Autodesk Fusion 360 part; units mm, degrees
(part 11 of 14)
  spline S137 degree 5 poles (-10.4982, 16.1129) (-10.4995, 16.1142) (-10.5054, 16.12) (-10.516, 16.1305) (-10.5314, 16.1454) (-10.5515, 16.1648) (-10.5752, 16.1872) (-10.5991, 16.2096) (-10.6232, 16.2317) (-10.6474, 16.2537) (-10.6718, 16.2756) (-10.6964, 16.2974) (-10.7212, 16.319) (-10.7461, 16.3405) (-10.7712, 16.3619) (-10.7965, 16.3832) (-10.8219, 16.4043) (-10.8474, 16.4253) (-10.8731, 16.4462) (-10.899, 16.4669) (-10.925, 16.4876) (-10.9511, 16.5081) (-10.9774, 16.5286) (-11.0038, 16.5489) (-11.0303, 16.5691) (-11.057, 16.5891) (-11.0838, 16.6091) (-11.1108, 16.629) (-11.1378, 16.6487) (-11.165, 16.6684) (-11.1924, 16.6879) (-11.2198, 16.7073) (-11.2474, 16.7267) (-11.2751, 16.7459) (-11.3029, 16.765) (-11.3308, 16.784) (-11.3589, 16.8029) (-11.387, 16.8217) (-11.4153, 16.8404) (-11.4437, 16.859) (-11.4722, 16.8775) (-11.5008, 16.8959) (-11.5295, 16.9142) (-11.5584, 16.9324) (-11.5873, 16.9505) (-11.6163, 16.9685) (-11.6455, 16.9864) (-11.6748, 17.0042) (-11.7041, 17.0219) (-11.7336, 17.0395) (-11.7632, 17.057) (-11.7928, 17.0744) (-11.8226, 17.0917) (-11.8525, 17.1089) (-11.8824, 17.126) (-11.9125, 17.143) (-11.9427, 17.1599) (-11.9729, 17.1768) (-11.9972, 17.1902) (-12.0155, 17.2001) (-12.0277, 17.2068) (-12.0338, 17.2101) knots 0.195913 0.195913 0.195913 0.195913 0.195913 0.195913 0.2 0.214286 0.228571 0.242857 0.257143 0.271429 0.285714 0.3 0.314286 0.328571 0.342857 0.357143 0.371429 0.385714 0.4 0.414286 0.428571 0.442857 0.457143 0.471429 0.485714 0.5 0.514286 0.528571 0.542857 0.557143 0.571429 0.585714 0.6 0.614286 0.628571 0.642857 0.657143 0.671429 0.685714 0.7 0.714286 0.728571 0.742857 0.757143 0.771429 0.785714 0.8 0.814286 0.828571 0.842857 0.857143 0.871429 0.885714 0.9 0.914286 0.928571 0.942857 0.957143 0.971429 0.985714 1 1 1 1 1 1
  arc A69 (-12.0338, 17.2101) -> (-12.6491, 16.763) centre (0, 0) ccw
  spline S138 degree 5 poles (-12.6491, 16.763) (-12.6479, 16.7562) (-12.6453, 16.7426) (-12.6415, 16.7221) (-12.6362, 16.6949) (-12.6296, 16.6609) (-12.6228, 16.627) (-12.6159, 16.5931) (-12.6089, 16.5593) (-12.6018, 16.5256) (-12.5945, 16.4919) (-12.5871, 16.4583) (-12.5796, 16.4248) (-12.572, 16.3913) (-12.5642, 16.3579) (-12.5563, 16.3246) (-12.5483, 16.2913) (-12.5402, 16.2582) (-12.5319, 16.225) (-12.5235, 16.192) (-12.515, 16.159) (-12.5064, 16.1261) (-12.4976, 16.0933) (-12.4887, 16.0606) (-12.4796, 16.0279) (-12.4704, 15.9953) (-12.4611, 15.9628) (-12.4517, 15.9303) (-12.4421, 15.898) (-12.4324, 15.8657) (-12.4225, 15.8335) (-12.4125, 15.8014) (-12.4024, 15.7694) (-12.3921, 15.7374) (-12.3817, 15.7056) (-12.3711, 15.6738) (-12.3604, 15.6422) (-12.3496, 15.6106) (-12.3385, 15.5791) (-12.3274, 15.5477) (-12.3161, 15.5164) (-12.3046, 15.4852) (-12.293, 15.4541) (-12.2813, 15.4231) (-12.2693, 15.3922) (-12.2573, 15.3614) (-12.245, 15.3307) (-12.2326, 15.3001) (-12.22, 15.2697) (-12.2073, 15.2393) (-12.1944, 15.2091) (-12.1813, 15.179) (-12.168, 15.149) (-12.1545, 15.1191) (-12.1409, 15.0894) (-12.1271, 15.0597) (-12.113, 15.0303) (-12.1008, 15.0051) (-12.0914, 14.9859) (-12.0847, 14.9726) (-12.081, 14.9651) (-12.0801, 14.9635) knots -1 -1 -1 -1 -1 -1 -0.985714 -0.971429 -0.957143 -0.942857 -0.928571 -0.914286 -0.9 -0.885714 -0.871429 -0.857143 -0.842857 -0.828571 -0.814286 -0.8 -0.785714 -0.771429 -0.757143 -0.742857 -0.728571 -0.714286 -0.7 -0.685714 -0.671429 -0.657143 -0.642857 -0.628571 -0.614286 -0.6 -0.585714 -0.571429 -0.557143 -0.542857 -0.528571 -0.514286 -0.5 -0.485714 -0.471429 -0.457143 -0.442857 -0.428571 -0.414286 -0.4 -0.385714 -0.371429 -0.357143 -0.342857 -0.328571 -0.314286 -0.3 -0.285714 -0.271429 -0.257143 -0.242857 -0.228571 -0.214286 -0.2 -0.195913 -0.195913 -0.195913 -0.195913 -0.195913 -0.195913
  spline S139 degree 3 poles (-12.203, 14.3578) (-12.1534, 14.4) (-12.1125, 14.4514) (-12.0527, 14.5671) (-12.0344, 14.6302) (-12.0247, 14.7411) (-12.027, 14.7875) (-12.0444, 14.8782) (-12.0594, 14.9222) (-12.0801, 14.9635) knots 0 0 0 0 0.019532 0.019532 0.039064 0.039064 0.052927 0.052927 0.06679 0.06679 0.06679 0.06679
  arc A70 (-12.203, 14.3578) -> (-12.2721, 14.2988) centre (0, 0) ccw
  spline S140 degree 3 poles (-12.8895, 14.2722) (-12.8366, 14.2342) (-12.7769, 14.2069) (-12.6502, 14.1767) (-12.5845, 14.1742) (-12.4745, 14.1914) (-12.4301, 14.2049) (-12.3462, 14.2436) (-12.3071, 14.2687) (-12.2721, 14.2988) knots 0 0 0 0 0.019532 0.019532 0.039064 0.039064 0.052927 0.052927 0.06679 0.06679 0.06679 0.06679
  spline S141 degree 5 poles (-12.8895, 14.2722) (-12.891, 14.2733) (-12.8978, 14.2782) (-12.9099, 14.2868) (-12.9274, 14.2992) (-12.9503, 14.3152) (-12.9772, 14.3336) (-13.0043, 14.3519) (-13.0316, 14.37) (-13.059, 14.388) (-13.0865, 14.4058) (-13.1142, 14.4234) (-13.1421, 14.4409) (-13.17, 14.4583) (-13.1982, 14.4755) (-13.2264, 14.4925) (-13.2548, 14.5094) (-13.2833, 14.5262) (-13.312, 14.5428) (-13.3408, 14.5592) (-13.3697, 14.5756) (-13.3987, 14.5918) (-13.4279, 14.6078) (-13.4571, 14.6237) (-13.4865, 14.6395) (-13.516, 14.6552) (-13.5456, 14.6707) (-13.5753, 14.6861) (-13.6051, 14.7014) (-13.6351, 14.7166) (-13.6651, 14.7316) (-13.6953, 14.7465) (-13.7255, 14.7612) (-13.7559, 14.7759) (-13.7863, 14.7904) (-13.8169, 14.8048) (-13.8476, 14.8191) (-13.8783, 14.8333) (-13.9092, 14.8473) (-13.9401, 14.8613) (-13.9712, 14.8751) (-14.0023, 14.8888) (-14.0335, 14.9023) (-14.0649, 14.9158) (-14.0963, 14.9291) (-14.1278, 14.9424) (-14.1594, 14.9555) (-14.1911, 14.9685) (-14.2228, 14.9814) (-14.2547, 14.9941) (-14.2866, 15.0068) (-14.3187, 15.0193) (-14.3508, 15.0318) (-14.383, 15.0441) (-14.4152, 15.0563) (-14.4476, 15.0684) (-14.4801, 15.0804) (-14.5126, 15.0923) (-14.5387, 15.1017) (-14.5583, 15.1087) (-14.5713, 15.1134) (-14.5779, 15.1157) knots 0.195913 0.195913 0.195913 0.195913 0.195913 0.195913 0.2 0.214286 0.228571 0.242857 0.257143 0.271429 0.285714 0.3 0.314286 0.328571 0.342857 0.357143 0.371429 0.385714 0.4 0.414286 0.428571 0.442857 0.457143 0.471429 0.485714 0.5 0.514286 0.528571 0.542857 0.557143 0.571429 0.585714 0.6 0.614286 0.628571 0.642857 0.657143 0.671429 0.685714 0.7 0.714286 0.728571 0.742857 0.757143 0.771429 0.785714 0.8 0.814286 0.828571 0.842857 0.857143 0.871429 0.885714 0.9 0.914286 0.928571 0.942857 0.957143 0.971429 0.985714 1 1 1 1 1 1
  arc A71 (-14.5779, 15.1157) -> (-15.1157, 14.5779) centre (0, 0) ccw
  spline S142 degree 5 poles (-15.1157, 14.5779) (-15.1134, 14.5713) (-15.1087, 14.5583) (-15.1017, 14.5387) (-15.0923, 14.5126) (-15.0804, 14.4801) (-15.0684, 14.4476) (-15.0563, 14.4152) (-15.0441, 14.383) (-15.0318, 14.3508) (-15.0193, 14.3187) (-15.0068, 14.2866) (-14.9941, 14.2547) (-14.9814, 14.2228) (-14.9685, 14.1911) (-14.9555, 14.1594) (-14.9424, 14.1278) (-14.9291, 14.0963) (-14.9158, 14.0649) (-14.9023, 14.0335) (-14.8888, 14.0023) (-14.8751, 13.9712) (-14.8613, 13.9401) (-14.8473, 13.9092) (-14.8333, 13.8783) (-14.8191, 13.8476) (-14.8048, 13.8169) (-14.7904, 13.7863) (-14.7759, 13.7559) (-14.7612, 13.7255) (-14.7465, 13.6953) (-14.7316, 13.6651) (-14.7166, 13.6351) (-14.7014, 13.6051) (-14.6861, 13.5753) (-14.6707, 13.5456) (-14.6552, 13.516) (-14.6395, 13.4865) (-14.6237, 13.4571) (-14.6078, 13.4279) (-14.5918, 13.3987) (-14.5756, 13.3697) (-14.5592, 13.3408) (-14.5428, 13.312) (-14.5262, 13.2833) (-14.5094, 13.2548) (-14.4925, 13.2264) (-14.4755, 13.1982) (-14.4583, 13.17) (-14.4409, 13.1421) (-14.4234, 13.1142) (-14.4058, 13.0865) (-14.388, 13.059) (-14.37, 13.0316) (-14.3519, 13.0043) (-14.3336, 12.9772) (-14.3152, 12.9503) (-14.2992, 12.9274) (-14.2868, 12.9099) (-14.2782, 12.8978) (-14.2733, 12.891) (-14.2722, 12.8895) knots -1 -1 -1 -1 -1 -1 -0.985714 -0.971429 -0.957143 -0.942857 -0.928571 -0.914286 -0.9 -0.885714 -0.871429 -0.857143 -0.842857 -0.828571 -0.814286 -0.8 -0.785714 -0.771429 -0.757143 -0.742857 -0.728571 -0.714286 -0.7 -0.685714 -0.671429 -0.657143 -0.642857 -0.628571 -0.614286 -0.6 -0.585714 -0.571429 -0.557143 -0.542857 -0.528571 -0.514286 -0.5 -0.485714 -0.471429 -0.457143 -0.442857 -0.428571 -0.414286 -0.4 -0.385714 -0.371429 -0.357143 -0.342857 -0.328571 -0.314286 -0.3 -0.285714 -0.271429 -0.257143 -0.242857 -0.228571 -0.214286 -0.2 -0.195913 -0.195913 -0.195913 -0.195913 -0.195913 -0.195913
  spline S143 degree 3 poles (-14.2988, 12.2721) (-14.2564, 12.3215) (-14.224, 12.3787) (-14.1831, 12.5023) (-14.1749, 12.5675) (-14.1826, 12.6785) (-14.1922, 12.724) (-14.2236, 12.8109) (-14.2452, 12.852) (-14.2722, 12.8895) knots 0 0 0 0 0.019532 0.019532 0.039064 0.039064 0.052927 0.052927 0.06679 0.06679 0.06679 0.06679
  arc A72 (-14.2988, 12.2721) -> (-14.3578, 12.203) centre (0, 0) ccw
  spline S144 degree 3 poles (-14.9635, 12.0801) (-14.9053, 12.0509) (-14.842, 12.0332) (-14.7122, 12.0233) (-14.6469, 12.031) (-14.541, 12.0652) (-14.4992, 12.0855) (-14.4224, 12.1369) (-14.3877, 12.1678) (-14.3578, 12.203) knots 0 0 0 0 0.019532 0.019532 0.039064 0.039064 0.052927 0.052927 0.06679 0.06679 0.06679 0.06679
  spline S145 degree 5 poles (-14.9635, 12.0801) (-14.9651, 12.081) (-14.9726, 12.0847) (-14.9859, 12.0914) (-15.0051, 12.1008) (-15.0303, 12.113) (-15.0597, 12.1271) (-15.0894, 12.1409) (-15.1191, 12.1545) (-15.149, 12.168) (-15.179, 12.1813) (-15.2091, 12.1944) (-15.2393, 12.2073) (-15.2697, 12.22) (-15.3001, 12.2326) (-15.3307, 12.245) (-15.3614, 12.2573) (-15.3922, 12.2693) (-15.4231, 12.2813) (-15.4541, 12.293) (-15.4852, 12.3046) (-15.5164, 12.3161) (-15.5477, 12.3274) (-15.5791, 12.3385) (-15.6106, 12.3496) (-15.6422, 12.3604) (-15.6738, 12.3711) (-15.7056, 12.3817) (-15.7374, 12.3921) (-15.7694, 12.4024) (-15.8014, 12.4125) (-15.8335, 12.4225) (-15.8657, 12.4324) (-15.898, 12.4421) (-15.9303, 12.4517) (-15.9628, 12.4611) (-15.9953, 12.4704) (-16.0279, 12.4796) (-16.0606, 12.4887) (-16.0933, 12.4976) (-16.1261, 12.5064) (-16.159, 12.515) (-16.192, 12.5235) (-16.225, 12.5319) (-16.2582, 12.5402) (-16.2913, 12.5483) (-16.3246, 12.5563) (-16.3579, 12.5642) (-16.3913, 12.572) (-16.4248, 12.5796) (-16.4583, 12.5871) (-16.4919, 12.5945) (-16.5256, 12.6018) (-16.5593, 12.6089) (-16.5931, 12.6159) (-16.627, 12.6228) (-16.6609, 12.6296) (-16.6949, 12.6362) (-16.7221, 12.6415) (-16.7426, 12.6453) (-16.7562, 12.6479) (-16.763, 12.6491) knots 0.195913 0.195913 0.195913 0.195913 0.195913 0.195913 0.2 0.214286 0.228571 0.242857 0.257143 0.271429 0.285714 0.3 0.314286 0.328571 0.342857 0.357143 0.371429 0.385714 0.4 0.414286 0.428571 0.442857 0.457143 0.471429 0.485714 0.5 0.514286 0.528571 0.542857 0.557143 0.571429 0.585714 0.6 0.614286 0.628571 0.642857 0.657143 0.671429 0.685714 0.7 0.714286 0.728571 0.742857 0.757143 0.771429 0.785714 0.8 0.814286 0.828571 0.842857 0.857143 0.871429 0.885714 0.9 0.914286 0.928571 0.942857 0.957143 0.971429 0.985714 1 1 1 1 1 1
  arc A73 (-16.763, 12.6491) -> (-17.2101, 12.0338) centre (0, 0) ccw
  spline S146 degree 5 poles (-17.2101, 12.0338) (-17.2068, 12.0277) (-17.2001, 12.0155) (-17.1902, 11.9972) (-17.1768, 11.9729) (-17.1599, 11.9427) (-17.143, 11.9125) (-17.126, 11.8824) (-17.1089, 11.8525) (-17.0917, 11.8226) (-17.0744, 11.7928) (-17.057, 11.7632) (-17.0395, 11.7336) (-17.0219, 11.7041) (-17.0042, 11.6748) (-16.9864, 11.6455) (-16.9685, 11.6163) (-16.9505, 11.5873) (-16.9324, 11.5584) (-16.9142, 11.5295) (-16.8959, 11.5008) (-16.8775, 11.4722) (-16.859, 11.4437) (-16.8404, 11.4153) (-16.8217, 11.387) (-16.8029, 11.3589) (-16.784, 11.3308) (-16.765, 11.3029) (-16.7459, 11.2751) (-16.7267, 11.2474) (-16.7073, 11.2198) (-16.6879, 11.1924) (-16.6684, 11.165) (-16.6487, 11.1378) (-16.629, 11.1108) (-16.6091, 11.0838) (-16.5891, 11.057) (-16.5691, 11.0303) (-16.5489, 11.0038) (-16.5286, 10.9774) (-16.5081, 10.9511) (-16.4876, 10.925) (-16.4669, 10.899) (-16.4462, 10.8731) (-16.4253, 10.8474) (-16.4043, 10.8219) (-16.3832, 10.7965) (-16.3619, 10.7712) (-16.3405, 10.7461) (-16.319, 10.7212) (-16.2974, 10.6964) (-16.2756, 10.6718) (-16.2537, 10.6474) (-16.2317, 10.6232) (-16.2096, 10.5991) (-16.1872, 10.5752) (-16.1648, 10.5515) (-16.1454, 10.5314) (-16.1305, 10.516) (-16.12, 10.5054) (-16.1142, 10.4995) (-16.1129, 10.4982) knots -1 -1 -1 -1 -1 -1 -0.985714 -0.971429 -0.957143 -0.942857 -0.928571 -0.914286 -0.9 -0.885714 -0.871429 -0.857143 -0.842857 -0.828571 -0.814286 -0.8 -0.785714 -0.771429 -0.757143 -0.742857 -0.728571 -0.714286 -0.7 -0.685714 -0.671429 -0.657143 -0.642857 -0.628571 -0.614286 -0.6 -0.585714 -0.571429 -0.557143 -0.542857 -0.528571 -0.514286 -0.5 -0.485714 -0.471429 -0.457143 -0.442857 -0.428571 -0.414286 -0.4 -0.385714 -0.371429 -0.357143 -0.342857 -0.328571 -0.314286 -0.3 -0.285714 -0.271429 -0.257143 -0.242857 -0.228571 -0.214286 -0.2 -0.195913 -0.195913 -0.195913 -0.195913 -0.195913 -0.195913
  spline S147 degree 3 poles (-16.0425, 9.8841) (-16.0084, 9.9396) (-15.9854, 10.0011) (-15.9643, 10.1296) (-15.9664, 10.1953) (-15.9914, 10.3038) (-16.008, 10.3472) (-16.0525, 10.4281) (-16.0803, 10.4653) (-16.1129, 10.4982) knots 0 0 0 0 0.019532 0.019532 0.039064 0.039064 0.052927 0.052927 0.06679 0.06679 0.06679 0.06679
  arc A74 (-16.0425, 9.8841) -> (-16.09, 9.8067) centre (0, 0) ccw
  spline S148 degree 3 poles (-16.669, 9.5906) (-16.607, 9.5708) (-16.5417, 9.5633) (-16.4119, 9.5737) (-16.3486, 9.5916) (-16.2494, 9.642) (-16.2113, 9.6685) (-16.1434, 9.7313) (-16.114, 9.7672) (-16.09, 9.8067) knots 0 0 0 0 0.019532 0.019532 0.039064 0.039064 0.052927 0.052927 0.06679 0.06679 0.06679 0.06679
  spline S149 degree 5 poles (-16.669, 9.5906) (-16.6708, 9.5912) (-16.6788, 9.5937) (-16.6929, 9.5982) (-16.7134, 9.6045) (-16.7401, 9.6127) (-16.7714, 9.6219) (-16.8028, 9.6309) (-16.8343, 9.6397) (-16.866, 9.6484) (-16.8977, 9.6568) (-16.9295, 9.665) (-16.9613, 9.673) (-16.9933, 9.6809) (-17.0254, 9.6885) (-17.0575, 9.696) (-17.0897, 9.7033) (-17.122, 9.7104) (-17.1544, 9.7174) (-17.1869, 9.7241) (-17.2194, 9.7307) (-17.252, 9.7372) (-17.2847, 9.7434) (-17.3175, 9.7495) (-17.3503, 9.7555) (-17.3832, 9.7613) (-17.4161, 9.7669) (-17.4492, 9.7723) (-17.4822, 9.7777) (-17.5154, 9.7828) (-17.5486, 9.7878) (-17.5819, 9.7927) (-17.6152, 9.7974) (-17.6486, 9.8019) (-17.6821, 9.8063) (-17.7156, 9.8106) (-17.7492, 9.8147) (-17.7828, 9.8187) (-17.8165, 9.8225) (-17.8502, 9.8262) (-17.884, 9.8297) (-17.9179, 9.8331) (-17.9518, 9.8364) (-17.9857, 9.8395) (-18.0197, 9.8425) (-18.0538, 9.8453) (-18.0879, 9.848) (-18.122, 9.8506) (-18.1562, 9.853) (-18.1905, 9.8553) (-18.2247, 9.8575) (-18.2591, 9.8595) (-18.2935, 9.8614) (-18.3279, 9.8632) (-18.3624, 9.8649) (-18.3969, 9.8664) (-18.4315, 9.8678) (-18.4661, 9.869) (-18.4938, 9.8699) (-18.5146, 9.8705) (-18.5285, 9.8709) (-18.5354, 9.8711) knots 0.195913 0.195913 0.195913 0.195913 0.195913 0.195913 0.2 0.214286 0.228571 0.242857 0.257143 0.271429 0.285714 0.3 0.314286 0.328571 0.342857 0.357143 0.371429 0.385714 0.4 0.414286 0.428571 0.442857 0.457143 0.471429 0.485714 0.5 0.514286 0.528571 0.542857 0.557143 0.571429 0.585714 0.6 0.614286 0.628571 0.642857 0.657143 0.671429 0.685714 0.7 0.714286 0.728571 0.742857 0.757143 0.771429 0.785714 0.8 0.814286 0.828571 0.842857 0.857143 0.871429 0.885714 0.9 0.914286 0.928571 0.942857 0.957143 0.971429 0.985714 1 1 1 1 1 1
  arc A75 (-18.5354, 9.8711) -> (-18.8807, 9.1934) centre (0, 0) ccw
  spline S150 degree 5 poles (-18.8807, 9.1934) (-18.8765, 9.1879) (-18.868, 9.1769) (-18.8553, 9.1604) (-18.8383, 9.1385) (-18.8169, 9.1112) (-18.7955, 9.0841) (-18.774, 9.0571) (-18.7524, 9.0301) (-18.7307, 9.0033) (-18.709, 8.9766) (-18.6871, 8.95) (-18.6652, 8.9236) (-18.6432, 8.8972) (-18.6211, 8.871) (-18.599, 8.8449) (-18.5768, 8.8189) (-18.5544, 8.793) (-18.532, 8.7672) (-18.5096, 8.7416) (-18.487, 8.7161) (-18.4644, 8.6907) (-18.4416, 8.6655) (-18.4188, 8.6403) (-18.3959, 8.6153) (-18.3729, 8.5905) (-18.3499, 8.5657) (-18.3267, 8.5411) (-18.3035, 8.5166) (-18.2802, 8.4923) (-18.2568, 8.4681) (-18.2333, 8.444) (-18.2098, 8.4201) (-18.1861, 8.3963) (-18.1623, 8.3726) (-18.1385, 8.3491) (-18.1146, 8.3258) (-18.0906, 8.3026) (-18.0665, 8.2795) (-18.0423, 8.2566) (-18.018, 8.2338) (-17.9936, 8.2112) (-17.9692, 8.1888) (-17.9446, 8.1665) (-17.92, 8.1444) (-17.8952, 8.1224) (-17.8704, 8.1006) (-17.8455, 8.079) (-17.8204, 8.0576) (-17.7953, 8.0364) (-17.77, 8.0153) (-17.7447, 7.9944) (-17.7192, 7.9737) (-17.6937, 7.9532) (-17.668, 7.9329) (-17.6423, 7.9127) (-17.6164, 7.8929) (-17.5941, 7.876) (-17.577, 7.8632) (-17.565, 7.8544) (-17.5582, 7.8494) (-17.5567, 7.8483) knots -1 -1 -1 -1 -1 -1 -0.985714 -0.971429 -0.957143 -0.942857 -0.928571 -0.914286 -0.9 -0.885714 -0.871429 -0.857143 -0.842857 -0.828571 -0.814286 -0.8 -0.785714 -0.771429 -0.757143 -0.742857 -0.728571 -0.714286 -0.7 -0.685714 -0.671429 -0.657143 -0.642857 -0.628571 -0.614286 -0.6 -0.585714 -0.571429 -0.557143 -0.542857 -0.528571 -0.514286 -0.5 -0.485714 -0.471429 -0.457143 -0.442857 -0.428571 -0.414286 -0.4 -0.385714 -0.371429 -0.357143 -0.342857 -0.328571 -0.314286 -0.3 -0.285714 -0.271429 -0.257143 -0.242857 -0.228571 -0.214286 -0.2 -0.195913 -0.195913 -0.195913 -0.195913 -0.195913 -0.195913
  spline S151 degree 3 poles (-17.3912, 7.2528) (-17.3662, 7.3129) (-17.3531, 7.3774) (-17.3523, 7.5076) (-17.3647, 7.5721) (-17.4064, 7.6753) (-17.4295, 7.7156) (-17.4862, 7.7886) (-17.5195, 7.821) (-17.5567, 7.8483) knots 0 0 0 0 0.019532 0.019532 0.039064 0.039064 0.052927 0.052927 0.06679 0.06679 0.06679 0.06679
  arc A76 (-17.3912, 7.2528) -> (-17.426, 7.1689) centre (0, 0) ccw
  spline S152 degree 3 poles (-17.9641, 6.8649) (-17.8997, 6.8551) (-17.8341, 6.8579) (-17.7075, 6.8885) (-17.6478, 6.916) (-17.5577, 6.9813) (-17.5242, 7.0135) (-17.467, 7.0861) (-17.4436, 7.1262) (-17.426, 7.1689) knots 0 0 0 0 0.019532 0.019532 0.039064 0.039064 0.052927 0.052927 0.06679 0.06679 0.06679 0.06679
  spline S153 degree 5 poles (-17.9641, 6.8649) (-17.9659, 6.8652) (-17.9742, 6.8665) (-17.9889, 6.8687) (-18.0101, 6.8717) (-18.0378, 6.8756) (-18.0701, 6.8798) (-18.1026, 6.8838) (-18.1351, 6.8876) (-18.1676, 6.8912) (-18.2003, 6.8945) (-18.233, 6.8977) (-18.2657, 6.9006) (-18.2985, 6.9033) (-18.3314, 6.9059) (-18.3643, 6.9083) (-18.3973, 6.9104) (-18.4303, 6.9124) (-18.4634, 6.9142) (-18.4965, 6.9158) (-18.5296, 6.9172) (-18.5629, 6.9185) (-18.5961, 6.9195) (-18.6294, 6.9205) (-18.6628, 6.9212) (-18.6962, 6.9218) (-18.7296, 6.9221) (-18.7631, 6.9224) (-18.7966, 6.9224) (-18.8301, 6.9224) (-18.8637, 6.9221) (-18.8973, 6.9217) (-18.931, 6.9211) (-18.9647, 6.9204) (-18.9984, 6.9195) (-19.0322, 6.9185) (-19.066, 6.9173) (-19.0998, 6.9159) (-19.1337, 6.9144) (-19.1676, 6.9128) (-19.2015, 6.911) (-19.2355, 6.9091) (-19.2695, 6.907) (-19.3035, 6.9048) (-19.3376, 6.9024) (-19.3716, 6.8999) (-19.4057, 6.8972) (-19.4399, 6.8944) (-19.474, 6.8915) (-19.5082, 6.8884) (-19.5424, 6.8852) (-19.5767, 6.8818) (-19.6109, 6.8783) (-19.6452, 6.8747) (-19.6795, 6.8709) (-19.7138, 6.867) (-19.7482, 6.863) (-19.7826, 6.8588) (-19.8101, 6.8553) (-19.8307, 6.8527) (-19.8445, 6.8509) (-19.8514, 6.85) knots 0.195913 0.195913 0.195913 0.195913 0.195913 0.195913 0.2 0.214286 0.228571 0.242857 0.257143 0.271429 0.285714 0.3 0.314286 0.328571 0.342857 0.357143 0.371429 0.385714 0.4 0.414286 0.428571 0.442857 0.457143 0.471429 0.485714 0.5 0.514286 0.528571 0.542857 0.557143 0.571429 0.585714 0.6 0.614286 0.628571 0.642857 0.657143 0.671429 0.685714 0.7 0.714286 0.728571 0.742857 0.757143 0.771429 0.785714 0.8 0.814286 0.828571 0.842857 0.857143 0.871429 0.885714 0.9 0.914286 0.928571 0.942857 0.957143 0.971429 0.985714 1 1 1 1 1 1
  arc A77 (-19.8514, 6.85) -> (-20.0864, 6.1266) centre (0, 0) ccw
  spline S154 degree 5 poles (-20.0864, 6.1266) (-20.0814, 6.1218) (-20.0713, 6.1123) (-20.0562, 6.098) (-20.0359, 6.079) (-20.0106, 6.0555) (-19.9851, 6.032) (-19.9597, 6.0087) (-19.9341, 5.9854) (-19.9085, 5.9623) (-19.8829, 5.9394) (-19.8571, 5.9165) (-19.8314, 5.8938) (-19.8055, 5.8712) (-19.7796, 5.8488) (-19.7536, 5.8265) (-19.7276, 5.8043) (-19.7015, 5.7822) (-19.6754, 5.7603) (-19.6492, 5.7385) (-19.6229, 5.7168) (-19.5966, 5.6953) (-19.5702, 5.6739) (-19.5437, 5.6526) (-19.5172, 5.6315) (-19.4906, 5.6105) (-19.4639, 5.5897) (-19.4372, 5.569) (-19.4105, 5.5485) (-19.3836, 5.5281) (-19.3567, 5.5078) (-19.3298, 5.4877) (-19.3027, 5.4678) (-19.2757, 5.448) (-19.2485, 5.4283) (-19.2213, 5.4088) (-19.194, 5.3895) (-19.1667, 5.3703) (-19.1393, 5.3513) (-19.1118, 5.3325) (-19.0842, 5.3138) (-19.0566, 5.2953) (-19.029, 5.277) (-19.0012, 5.2588) (-18.9734, 5.2408) (-18.9455, 5.223) (-18.9176, 5.2054) (-18.8896, 5.1879) (-18.8615, 5.1707) (-18.8333, 5.1536) (-18.8051, 5.1368) (-18.7768, 5.1201) (-18.7485, 5.1036) (-18.72, 5.0873) (-18.6915, 5.0713) (-18.6629, 5.0555) (-18.6342, 5.0399) (-18.6096, 5.0267) (-18.5906, 5.0168) (-18.5774, 5.0099) (-18.57, 5.006) (-18.5683, 5.0052) knots -1 -1 -1 -1 -1 -1 -0.985714 -0.971429 -0.957143 -0.942857 -0.928571 -0.914286 -0.9 -0.885714 -0.871429 -0.857143 -0.842857 -0.828571 -0.814286 -0.8 -0.785714 -0.771429 -0.757143 -0.742857 -0.728571 -0.714286 -0.7 -0.685714 -0.671429 -0.657143 -0.642857 -0.628571 -0.614286 -0.6 -0.585714 -0.571429 -0.557143 -0.542857 -0.528571 -0.514286 -0.5 -0.485714 -0.471429 -0.457143 -0.442857 -0.428571 -0.414286 -0.4 -0.385714 -0.371429 -0.357143 -0.342857 -0.328571 -0.314286 -0.3 -0.285714 -0.271429 -0.257143 -0.242857 -0.228571 -0.214286 -0.2 -0.195913 -0.195913 -0.195913 -0.195913 -0.195913 -0.195913
  spline S155 degree 3 poles (-18.3117, 4.443) (-18.2964, 4.5062) (-18.2935, 4.5719) (-18.3131, 4.7006) (-18.3354, 4.7625) (-18.3928, 4.8579) (-18.4219, 4.894) (-18.4893, 4.9572) (-18.5273, 4.984) (-18.5683, 5.0052) knots 0 0 0 0 0.019532 0.019532 0.039064 0.039064 0.052927 0.052927 0.06679 0.06679 0.06679 0.06679
  arc A78 (-18.3117, 4.443) -> (-18.3329, 4.3546) centre (0, 0) ccw
  spline S156 degree 3 poles (-18.8168, 3.9702) (-18.7517, 3.9705) (-18.6873, 3.9836) (-18.5671, 4.0336) (-18.5124, 4.0701) (-18.4336, 4.1487) (-18.4056, 4.1858) (-18.3605, 4.2664) (-18.3436, 4.3097) (-18.3329, 4.3546) knots 0 0 0 0 0.019532 0.019532 0.039064 0.039064 0.052927 0.052927 0.06679 0.06679 0.06679 0.06679
  spline S157 degree 5 poles (-18.8168, 3.9702) (-18.8187, 3.9702) (-18.8271, 3.9701) (-18.8419, 3.97) (-18.8633, 3.9697) (-18.8913, 3.9692) (-18.9239, 3.9683) (-18.9566, 3.9672) (-18.9893, 3.9658) (-19.022, 3.9643) (-19.0547, 3.9625) (-19.0875, 3.9605) (-19.1203, 3.9583) (-19.1532, 3.9558) (-19.186, 3.9532) (-19.2189, 3.9504) (-19.2518, 3.9474) (-19.2847, 3.9442) (-19.3177, 3.9407) (-19.3506, 3.9372) (-19.3836, 3.9334) (-19.4166, 3.9294) (-19.4496, 3.9253) (-19.4827, 3.921) (-19.5157, 3.9165) (-19.5488, 3.9118) (-19.5819, 3.907) (-19.615, 3.902) (-19.6481, 3.8968) (-19.6812, 3.8914) (-19.7143, 3.8859) (-19.7475, 3.8803) (-19.7806, 3.8744) (-19.8138, 3.8684) (-19.847, 3.8623) (-19.8802, 3.856) (-19.9134, 3.8495) (-19.9466, 3.8429) (-19.9798, 3.8361) (-20.013, 3.8292) (-20.0463, 3.8221) (-20.0795, 3.8149) (-20.1127, 3.8075) (-20.146, 3.8) (-20.1793, 3.7923) (-20.2125, 3.7845) (-20.2458, 3.7766) (-20.2791, 3.7685) (-20.3123, 3.7602) (-20.3456, 3.7518) (-20.3789, 3.7433) (-20.4122, 3.7346) (-20.4455, 3.7258) (-20.4788, 3.7168) (-20.5121, 3.7078) (-20.5454, 3.6985) (-20.5787, 3.6892) (-20.612, 3.6797) (-20.6386, 3.6719) (-20.6586, 3.6661) (-20.6719, 3.6622) (-20.6786, 3.6602) knots 0.195913 0.195913 0.195913 0.195913 0.195913 0.195913 0.2 0.214286 0.228571 0.242857 0.257143 0.271429 0.285714 0.3 0.314286 0.328571 0.342857 0.357143 0.371429 0.385714 0.4 0.414286 0.428571 0.442857 0.457143 0.471429 0.485714 0.5 0.514286 0.528571 0.542857 0.557143 0.571429 0.585714 0.6 0.614286 0.628571 0.642857 0.657143 0.671429 0.685714 0.7 0.714286 0.728571 0.742857 0.757143 0.771429 0.785714 0.8 0.814286 0.828571 0.842857 0.857143 0.871429 0.885714 0.9 0.914286 0.928571 0.942857 0.957143 0.971429 0.985714 1 1 1 1 1 1
  arc A79 (-20.6786, 3.6602) -> (-20.7975, 2.909) centre (0, 0) ccw
  spline S158 degree 5 poles (-20.7975, 2.909) (-20.7918, 2.905) (-20.7804, 2.8972) (-20.7632, 2.8854) (-20.7402, 2.8699) (-20.7115, 2.8506) (-20.6827, 2.8314) (-20.6539, 2.8123) (-20.625, 2.7934) (-20.5961, 2.7746) (-20.5672, 2.7559) (-20.5382, 2.7374) (-20.5092, 2.719) (-20.4801, 2.7007) (-20.451, 2.6826) (-20.4219, 2.6646) (-20.3927, 2.6467) (-20.3635, 2.629) (-20.3342, 2.6114) (-20.3049, 2.594) (-20.2756, 2.5767) (-20.2462, 2.5596) (-20.2168, 2.5426) (-20.1873, 2.5257) (-20.1578, 2.509) (-20.1283, 2.4925) (-20.0987, 2.476) (-20.0691, 2.4598) (-20.0395, 2.4437) (-20.0098, 2.4277) (-19.98, 2.4119) (-19.9503, 2.3963) (-19.9204, 2.3808) (-19.8906, 2.3655) (-19.8607, 2.3504) (-19.8308, 2.3354) (-19.8008, 2.3206) (-19.7708, 2.3059) (-19.7408, 2.2914) (-19.7107, 2.2771) (-19.6805, 2.263) (-19.6504, 2.249) (-19.6202, 2.2352) (-19.5899, 2.2216) (-19.5597, 2.2082) (-19.5293, 2.195) (-19.499, 2.1819) (-19.4686, 2.1691) (-19.4382, 2.1564) (-19.4077, 2.144) (-19.3772, 2.1317) (-19.3466, 2.1197) (-19.316, 2.1079) (-19.2854, 2.0963) (-19.2547, 2.0849) (-19.224, 2.0737) (-19.1932, 2.0628) (-19.1668, 2.0536) (-19.1465, 2.0468) (-19.1324, 2.0421) (-19.1245, 2.0394) (-19.1227, 2.0388) knots -1 -1 -1 -1 -1 -1 -0.985714 -0.971429 -0.957143 -0.942857 -0.928571 -0.914286 -0.9 -0.885714 -0.871429 -0.857143 -0.842857 -0.828571 -0.814286 -0.8 -0.785714 -0.771429 -0.757143 -0.742857 -0.728571 -0.714286 -0.7 -0.685714 -0.671429 -0.657143 -0.642857 -0.628571 -0.614286 -0.6 -0.585714 -0.571429 -0.557143 -0.542857 -0.528571 -0.514286 -0.5 -0.485714 -0.471429 -0.457143 -0.442857 -0.428571 -0.414286 -0.4 -0.385714 -0.371429 -0.357143 -0.342857 -0.328571 -0.314286 -0.3 -0.285714 -0.271429 -0.257143 -0.242857 -0.228571 -0.214286 -0.2 -0.195913 -0.195913 -0.195913 -0.195913 -0.195913 -0.195913
  spline S159 degree 3 poles (-18.7813, 1.5237) (-18.776, 1.5886) (-18.7835, 1.6539) (-18.823, 1.7779) (-18.8547, 1.8355) (-18.9263, 1.9208) (-18.9607, 1.9519) (-19.0372, 2.0038) (-19.0788, 2.0243) (-19.1227, 2.0388) knots 0 0 0 0 0.019532 0.019532 0.039064 0.039064 0.052927 0.052927 0.06679 0.06679 0.06679 0.06679
  circle A80 centre (0, 0) radius 2
  line L0 (1.3229, -1.5) -> (-1.3229, -1.5)
  constraint coincident A80 L0.start
  constraint coincident A80 L0.end
extrude "Extrude11" add sketch "Sketch16" against normal blind 5 contours A80 L0 picked at (-0.3643, -1.5583)
named bodies: "Spur Gear (40 teeth)"

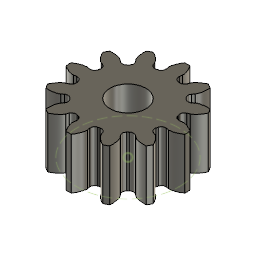
design "stopping mechanism small gear"
description: Spur Gear; Module: 1.0; Num Teeth: 12; Pressure Angle: 20.0; Backlash: 0.00 mm
part number: 2026-03-18-22-21-27-234
Autodesk Fusion 360 part; units mm, degrees
sketch "Base Circle" plane through (0, 0, 0) normal (0, 0, 1) x (1, 0, 0)
  circle A0 centre (0, 0) radius 4.843
  circle A1 centre (0, 0) radius 2.1
extrude "Extrude1" add sketch "Base Circle" along normal blind 6
sketch "Gear Tooth" plane through (0, 0, 0) normal (0, 0, 1) x (1, 0, 0)
  spline S0 degree 5 poles (5.5783, -0.8192) (5.5823, -0.8197) (5.5902, -0.8208) (5.6021, -0.822) (5.6181, -0.8228) (5.6381, -0.8229) (5.6583, -0.8223) (5.6784, -0.8212) (5.6986, -0.8199) (5.7188, -0.8184) (5.7391, -0.8168) (5.7593, -0.8149) (5.7796, -0.8127) (5.7999, -0.8102) (5.8203, -0.8073) (5.8406, -0.8041) (5.861, -0.8006) (5.8814, -0.7969) (5.9018, -0.793) (5.9222, -0.7888) (5.9426, -0.7845) (5.9631, -0.7799) (5.9835, -0.7752) (6.0039, -0.7702) (6.0244, -0.765) (6.0448, -0.7596) (6.0653, -0.7539) (6.0857, -0.7481) (6.1061, -0.7421) (6.1266, -0.7359) (6.147, -0.7295) (6.1675, -0.7229) (6.1879, -0.7161) (6.2083, -0.7092) (6.2288, -0.7021) (6.2492, -0.6947) (6.2696, -0.6873) (6.29, -0.6796) (6.3104, -0.6717) (6.3308, -0.6637) (6.3512, -0.6555) (6.3715, -0.6472) (6.3919, -0.6387) (6.4122, -0.63) (6.4325, -0.6211) (6.4528, -0.6121) (6.4731, -0.6029) (6.4934, -0.5936) (6.5137, -0.5841) (6.5339, -0.5744) (6.5541, -0.5646) (6.5743, -0.5546) (6.5945, -0.5445) (6.6147, -0.5342) (6.6348, -0.5238) (6.655, -0.5132) (6.6751, -0.5024) (6.6951, -0.4915) (6.7152, -0.4805) (6.7352, -0.4693) (6.7552, -0.4579) (6.7752, -0.4464) (6.7952, -0.4348) (6.8151, -0.423) (6.835, -0.4111) (6.8549, -0.399) (6.8747, -0.3867) (6.8945, -0.3744) (6.9143, -0.3619) (6.9341, -0.3492) (6.9538, -0.3364) (6.9695, -0.3261) (6.9813, -0.3182) (6.9892, -0.313) (6.9931, -0.3103) knots 0 0 0 0 0 0 0.01428571 0.02857143 0.04285714 0.05714286 0.07142857 0.08571429 0.1 0.11428571 0.12857143 0.14285714 0.15714286 0.17142857 0.18571429 0.2 0.21428571 0.22857143 0.24285714 0.25714286 0.27142857 0.28571429 0.3 0.31428571 0.32857143 0.34285714 0.35714286 0.37142857 0.38571429 0.4 0.41428571 0.42857143 0.44285714 0.45714286 0.47142857 0.48571429 0.5 0.51428571 0.52857143 0.54285714 0.55714286 0.57142857 0.58571429 0.6 0.61428571 0.62857143 0.64285714 0.65714286 0.67142857 0.68571429 0.7 0.71428571 0.72857143 0.74285714 0.75714286 0.77142857 0.78571429 0.8 0.81428571 0.82857143 0.84285714 0.85714286 0.87142857 0.88571429 0.9 0.91428571 0.92857143 0.94285714 0.95714286 0.97142857 0.98571429 1 1 1 1 1 1
  spline S1 degree 5 poles (5.5783, 0.8192) (5.5823, 0.8197) (5.5902, 0.8208) (5.6021, 0.822) (5.6181, 0.8228) (5.6381, 0.8229) (5.6583, 0.8223) (5.6784, 0.8212) (5.6986, 0.8199) (5.7188, 0.8184) (5.7391, 0.8168) (5.7593, 0.8149) (5.7796, 0.8127) (5.7999, 0.8102) (5.8203, 0.8073) (5.8406, 0.8041) (5.861, 0.8006) (5.8814, 0.7969) (5.9018, 0.793) (5.9222, 0.7888) (5.9426, 0.7845) (5.9631, 0.7799) (5.9835, 0.7752) (6.0039, 0.7702) (6.0244, 0.765) (6.0448, 0.7596) (6.0653, 0.7539) (6.0857, 0.7481) (6.1061, 0.7421) (6.1266, 0.7359) (6.147, 0.7295) (6.1675, 0.7229) (6.1879, 0.7161) (6.2083, 0.7092) (6.2288, 0.7021) (6.2492, 0.6947) (6.2696, 0.6873) (6.29, 0.6796) (6.3104, 0.6717) (6.3308, 0.6637) (6.3512, 0.6555) (6.3715, 0.6472) (6.3919, 0.6387) (6.4122, 0.63) (6.4325, 0.6211) (6.4528, 0.6121) (6.4731, 0.6029) (6.4934, 0.5936) (6.5137, 0.5841) (6.5339, 0.5744) (6.5541, 0.5646) (6.5743, 0.5546) (6.5945, 0.5445) (6.6147, 0.5342) (6.6348, 0.5238) (6.655, 0.5132) (6.6751, 0.5024) (6.6951, 0.4915) (6.7152, 0.4805) (6.7352, 0.4693) (6.7552, 0.4579) (6.7752, 0.4464) (6.7952, 0.4348) (6.8151, 0.423) (6.835, 0.4111) (6.8549, 0.399) (6.8747, 0.3867) (6.8945, 0.3744) (6.9143, 0.3619) (6.9341, 0.3492) (6.9538, 0.3364) (6.9695, 0.3261) (6.9813, 0.3182) (6.9892, 0.313) (6.9931, 0.3103) knots 0 0 0 0 0 0 0.01428571 0.02857143 0.04285714 0.05714286 0.07142857 0.08571429 0.1 0.11428571 0.12857143 0.14285714 0.15714286 0.17142857 0.18571429 0.2 0.21428571 0.22857143 0.24285714 0.25714286 0.27142857 0.28571429 0.3 0.31428571 0.32857143 0.34285714 0.35714286 0.37142857 0.38571429 0.4 0.41428571 0.42857143 0.44285714 0.45714286 0.47142857 0.48571429 0.5 0.51428571 0.52857143 0.54285714 0.55714286 0.57142857 0.58571429 0.6 0.61428571 0.62857143 0.64285714 0.65714286 0.67142857 0.68571429 0.7 0.71428571 0.72857143 0.74285714 0.75714286 0.77142857 0.78571429 0.8 0.81428571 0.82857143 0.84285714 0.85714286 0.87142857 0.88571429 0.9 0.91428571 0.92857143 0.94285714 0.95714286 0.97142857 0.98571429 1 1 1 1 1 1
  arc A0 (6.9931, -0.3103) -> (6.9931, 0.3103) centre (0, 0) ccw
  line L0 (4.7817, -0.7022) -> (5.5783, -0.8192)
  line L1 (4.7817, 0.7022) -> (5.5783, 0.8192)
  line L2 (4.7817, -0.7022) -> (4.7817, 0.7022)
  point P0 (5.6763, -0.8213)
  point P1 (5.7758, -0.8131)
  point P2 (5.8761, -0.7978)
  point P3 (5.977, -0.7767)
  point P4 (6.0784, -0.7502)
  point P5 (6.1802, -0.7187)
  point P6 (6.2821, -0.6825)
  point P7 (6.3842, -0.6419)
  point P8 (6.4862, -0.5969)
  point P9 (6.5882, -0.5477)
  point P10 (6.6899, -0.4943)
  point P11 (6.7914, -0.437)
  point P12 (6.8925, -0.3756)
  point P13 (5.6763, 0.8213)
  point P14 (5.7758, 0.8131)
  point P15 (5.8761, 0.7978)
  point P16 (5.977, 0.7767)
  point P17 (6.0784, 0.7502)
  point P18 (6.1802, 0.7187)
  point P19 (6.2821, 0.6825)
  point P20 (6.3842, 0.6419)
  point P21 (6.4862, 0.5969)
  point P22 (6.5882, 0.5477)
  point P23 (6.6899, 0.4943)
  point P24 (6.7914, 0.437)
  point P25 (6.8925, 0.3756)
extrude "Extrude2" add sketch "Gear Tooth" along normal blind 6
fillet "Fillet1" radius 0.5 2 edges at (4.7916, -0.7036, 3) (4.7916, 0.7036, 3)
pattern_circular "C-Pattern1" count 12 over 360 about axis through (0, 0, 0) along (0, 0, 1) of "Extrude2", "Fillet1"
sketch "Diametrial Pitch Circle" plane through (0, 0, 0) normal (0, 0, 1) x (1, 0, 0)
  circle A0 centre (0, 0) radius 6 construction
named bodies: "Spur Gear (12 teeth)"

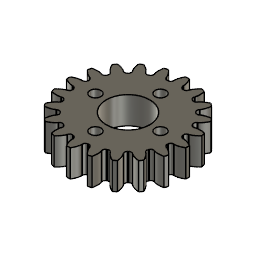
design "Smaller Gear"
description: Spur Gear; Module: 1.0; Num Teeth: 30; Pressure Angle: 20.0; Backlash: 0.00 mm
part number: 2026-02-09-12-11-18-481
Autodesk Fusion 360 part; units mm, degrees
sketch "Base Circle" plane through (0, 0, 0) normal (0, 0, 1) x (1, 0, 0)
  circle A0 centre (0, 0) radius 8.843
  circle A1 centre (0, 0) radius 4
extrude "Extrude5" add sketch "Base Circle" along normal blind 5
sketch "Gear Tooth" plane through (0, 0, 0) normal (0, 0, 1) x (1, 0, 0)
  spline S0 degree 5 poles (9.3559, -0.8768) (9.3606, -0.8772) (9.3699, -0.878) (9.3839, -0.8788) (9.4026, -0.8791) (9.426, -0.8785) (9.4495, -0.8772) (9.473, -0.8755) (9.4965, -0.8735) (9.52, -0.8714) (9.5435, -0.8691) (9.567, -0.8666) (9.5906, -0.8638) (9.6142, -0.8607) (9.6377, -0.8572) (9.6613, -0.8535) (9.6849, -0.8494) (9.7085, -0.8451) (9.7321, -0.8406) (9.7557, -0.836) (9.7793, -0.8311) (9.8029, -0.8261) (9.8265, -0.8208) (9.8501, -0.8153) (9.8737, -0.8096) (9.8973, -0.8037) (9.9209, -0.7977) (9.9445, -0.7914) (9.968, -0.7849) (9.9916, -0.7783) (10.0152, -0.7715) (10.0388, -0.7645) (10.0623, -0.7574) (10.0859, -0.7501) (10.1095, -0.7426) (10.133, -0.7349) (10.1565, -0.7271) (10.1801, -0.7191) (10.2036, -0.711) (10.2271, -0.7027) (10.2506, -0.6942) (10.2741, -0.6856) (10.2976, -0.6768) (10.321, -0.6679) (10.3445, -0.6588) (10.3679, -0.6496) (10.3913, -0.6402) (10.4148, -0.6307) (10.4382, -0.621) (10.4615, -0.6112) (10.4849, -0.6013) (10.5083, -0.5912) (10.5316, -0.5809) (10.5549, -0.5705) (10.5782, -0.56) (10.6015, -0.5493) (10.6248, -0.5385) (10.6481, -0.5276) (10.6713, -0.5165) (10.6945, -0.5053) (10.7177, -0.4939) (10.7409, -0.4824) (10.7641, -0.4708) (10.7872, -0.4591) (10.8103, -0.4472) (10.8334, -0.4352) (10.8565, -0.423) (10.8796, -0.4107) (10.9026, -0.3983) (10.9256, -0.3858) (10.9486, -0.3731) (10.967, -0.3629) (10.9807, -0.3552) (10.9899, -0.35) (10.9945, -0.3474) knots 0 0 0 0 0 0 0.01428571 0.02857143 0.04285714 0.05714286 0.07142857 0.08571429 0.1 0.11428571 0.12857143 0.14285714 0.15714286 0.17142857 0.18571429 0.2 0.21428571 0.22857143 0.24285714 0.25714286 0.27142857 0.28571429 0.3 0.31428571 0.32857143 0.34285714 0.35714286 0.37142857 0.38571429 0.4 0.41428571 0.42857143 0.44285714 0.45714286 0.47142857 0.48571429 0.5 0.51428571 0.52857143 0.54285714 0.55714286 0.57142857 0.58571429 0.6 0.61428571 0.62857143 0.64285714 0.65714286 0.67142857 0.68571429 0.7 0.71428571 0.72857143 0.74285714 0.75714286 0.77142857 0.78571429 0.8 0.81428571 0.82857143 0.84285714 0.85714286 0.87142857 0.88571429 0.9 0.91428571 0.92857143 0.94285714 0.95714286 0.97142857 0.98571429 1 1 1 1 1 1
  spline S1 degree 5 poles (9.3559, 0.8768) (9.3606, 0.8772) (9.3699, 0.878) (9.3839, 0.8788) (9.4026, 0.8791) (9.426, 0.8785) (9.4495, 0.8772) (9.473, 0.8755) (9.4965, 0.8735) (9.52, 0.8714) (9.5435, 0.8691) (9.567, 0.8666) (9.5906, 0.8638) (9.6142, 0.8607) (9.6377, 0.8572) (9.6613, 0.8535) (9.6849, 0.8494) (9.7085, 0.8451) (9.7321, 0.8406) (9.7557, 0.836) (9.7793, 0.8311) (9.8029, 0.8261) (9.8265, 0.8208) (9.8501, 0.8153) (9.8737, 0.8096) (9.8973, 0.8037) (9.9209, 0.7977) (9.9445, 0.7914) (9.968, 0.7849) (9.9916, 0.7783) (10.0152, 0.7715) (10.0388, 0.7645) (10.0623, 0.7574) (10.0859, 0.7501) (10.1095, 0.7426) (10.133, 0.7349) (10.1565, 0.7271) (10.1801, 0.7191) (10.2036, 0.711) (10.2271, 0.7027) (10.2506, 0.6942) (10.2741, 0.6856) (10.2976, 0.6768) (10.321, 0.6679) (10.3445, 0.6588) (10.3679, 0.6496) (10.3913, 0.6402) (10.4148, 0.6307) (10.4382, 0.621) (10.4615, 0.6112) (10.4849, 0.6013) (10.5083, 0.5912) (10.5316, 0.5809) (10.5549, 0.5705) (10.5782, 0.56) (10.6015, 0.5493) (10.6248, 0.5385) (10.6481, 0.5276) (10.6713, 0.5165) (10.6945, 0.5053) (10.7177, 0.4939) (10.7409, 0.4824) (10.7641, 0.4708) (10.7872, 0.4591) (10.8103, 0.4472) (10.8334, 0.4352) (10.8565, 0.423) (10.8796, 0.4107) (10.9026, 0.3983) (10.9256, 0.3858) (10.9486, 0.3731) (10.967, 0.3629) (10.9807, 0.3552) (10.9899, 0.35) (10.9945, 0.3474) knots 0 0 0 0 0 0 0.01428571 0.02857143 0.04285714 0.05714286 0.07142857 0.08571429 0.1 0.11428571 0.12857143 0.14285714 0.15714286 0.17142857 0.18571429 0.2 0.21428571 0.22857143 0.24285714 0.25714286 0.27142857 0.28571429 0.3 0.31428571 0.32857143 0.34285714 0.35714286 0.37142857 0.38571429 0.4 0.41428571 0.42857143 0.44285714 0.45714286 0.47142857 0.48571429 0.5 0.51428571 0.52857143 0.54285714 0.55714286 0.57142857 0.58571429 0.6 0.61428571 0.62857143 0.64285714 0.65714286 0.67142857 0.68571429 0.7 0.71428571 0.72857143 0.74285714 0.75714286 0.77142857 0.78571429 0.8 0.81428571 0.82857143 0.84285714 0.85714286 0.87142857 0.88571429 0.9 0.91428571 0.92857143 0.94285714 0.95714286 0.97142857 0.98571429 1 1 1 1 1 1
  arc A0 (10.9945, -0.3474) -> (10.9945, 0.3474) centre (0, 0) ccw
  line L0 (8.7945, -0.8242) -> (9.3559, -0.8768)
  line L1 (8.7945, 0.8242) -> (9.3559, 0.8768)
  line L2 (8.7945, -0.8242) -> (8.7945, 0.8242)
  point P0 (9.471, -0.8756)
  point P1 (9.5871, -0.8642)
  point P2 (9.7036, -0.846)
  point P3 (9.8206, -0.8221)
  point P4 (9.9379, -0.7931)
  point P5 (10.0553, -0.7595)
  point P6 (10.1729, -0.7215)
  point P7 (10.2906, -0.6794)
  point P8 (10.4082, -0.6333)
  point P9 (10.5258, -0.5834)
  point P10 (10.6433, -0.5298)
  point P11 (10.7606, -0.4725)
  point P12 (10.8777, -0.4117)
  point P13 (9.471, 0.8756)
  point P14 (9.5871, 0.8642)
  point P15 (9.7036, 0.846)
  point P16 (9.8206, 0.8221)
  point P17 (9.9379, 0.7931)
  point P18 (10.0553, 0.7595)
  point P19 (10.1729, 0.7215)
  point P20 (10.2906, 0.6794)
  point P21 (10.4082, 0.6333)
  point P22 (10.5258, 0.5834)
  point P23 (10.6433, 0.5298)
  point P24 (10.7606, 0.4725)
  point P25 (10.8777, 0.4117)
extrude "Extrude6" add sketch "Gear Tooth" along normal blind 5
fillet "Fillet3" radius 0.5 2 edges at (8.8044, -0.8251, 2.5) (8.8044, 0.8251, 2.5)
pattern_circular "C-Pattern3" count 20 over 360 about axis through (0, 0, 0) along (0, 0, 1) of "Extrude6", "Fillet3"
sketch "Diametrial Pitch Circle" plane through (0, 0, 0) normal (0, 0, 1) x (1, 0, 0)
  circle A0 centre (0, 0) radius 10 construction